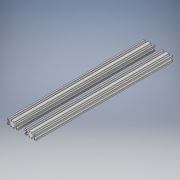
# Autodesk Inventor part: Rail
Saved by Autodesk Inventor 2019 (Build 230136000, 136)
## iProperties
Created: 2021-06-17
Part Number: Rail
Material: Generic
Document SubType Name: Modeling
Designer: 91742
Density: 1 g/cm^3
Appearance: Default
Author: 91742
Autodesk Inventor part; units mm, degrees
ref_plane "YZ Plane" through (0, 0, 0) normal (1, 0, 0) x (0, 1, 0)
ref_plane "XZ Plane" through (0, 0, 0) normal (0, 1, 0) x (-1, 0, 0)
ref_plane "XY Plane" through (0, 0, 0) normal (0, 0, 1) x (1, 0, 0)
sketch "Sketch1" plane through (0, 0, 0) normal (0, 0, 1) x (1, 0, 0)
  circle A0 centre (10, 0) radius 2.1
  line L0 (14.5874, 9.8723) -> (19.0874, 9.8723)
  line L1 (19.0874, 9.8723) -> (14.5874, 9.8723)
  line L2 (14.5874, 9.8723) -> (13.5268, 8.8116)
  line L3 (14.5874, 9.8723) -> (16.0874, 9.8723) construction
  line L4 (13.5268, 8.8116) -> (15.9268, 8.8116)
  line L5 (6.9, 0) -> (6.9, 1.8336)
  line L6 (15.9268, 6.8867) -> (13.1, 4.0599)
  line L7 (15.9268, 8.8116) -> (15.9268, 6.8867)
  line L8 (20.1068, 8.8259) -> (20.1068, 4.3259)
  line L9 (20.1068, 4.3259) -> (19.0461, 3.2652)
  line L10 (19.0461, 3.2652) -> (19.0461, 5.6652)
  line L11 (13.1, 1.8336) -> (16.9316, 5.6652)
  line L12 (19.0461, 5.6652) -> (16.9316, 5.6652)
  line L13 (13.1, 4.0599) -> (6.9, 4.0599)
  line L14 (5.4128, 9.8723) -> (0.9128, 9.8723)
  line L15 (0.9128, 9.8723) -> (5.4128, 9.8723)
  line L16 (5.4128, 9.8723) -> (6.4735, 8.8116)
  line L17 (5.4128, 9.8723) -> (3.9128, 9.8723) construction
  line L18 (4.0732, 6.8867) -> (6.9, 4.0599)
  line L19 (4.0732, 8.8116) -> (4.0732, 6.8867)
  line L20 (6.9, 1.8336) -> (3.0684, 5.6652)
  line L21 (13.1, 0) -> (13.1, 1.8336)
  line L22 (3.0684, 5.6652) -> (3.0684, 8.8116)
  line L23 (3.0684, 8.8116) -> (0.9126, 8.8116)
  circle A1 centre (10, 0) radius 2.1
  line L24 (14.5874, -9.8723) -> (19.0874, -9.8723)
  line L25 (19.0874, -9.8723) -> (14.5874, -9.8723)
  line L26 (14.5874, -9.8723) -> (13.5268, -8.8116)
  line L27 (14.5874, -9.8723) -> (16.0874, -9.8723) construction
  line L28 (13.5268, -8.8116) -> (15.9268, -8.8116)
  line L29 (6.9, 0) -> (6.9, -1.8336)
  line L30 (15.9268, -6.8867) -> (13.1, -4.0599)
  line L31 (15.9268, -8.8116) -> (15.9268, -6.8867)
  line L32 (20.1068, -8.8259) -> (20.1068, -4.3259)
  line L33 (20.1068, -4.3259) -> (19.0461, -3.2652)
  line L34 (19.0461, -3.2652) -> (19.0461, -5.6652)
  line L35 (13.1, -1.8336) -> (16.9316, -5.6652)
  line L36 (19.0461, -5.6652) -> (16.9316, -5.6652)
  line L37 (13.1, -4.0599) -> (6.9, -4.0599)
  line L38 (5.4126, -9.8723) -> (0.9126, -9.8723)
  line L39 (0.9126, -9.8723) -> (5.4126, -9.8723)
  line L40 (5.4126, -9.8723) -> (3.9126, -9.8723) construction
  line L41 (4.0732, -8.8116) -> (4.0732, -6.8867)
  line L42 (6.4732, -8.8116) -> (4.0732, -8.8116)
  line L43 (5.4126, -9.8723) -> (6.4732, -8.8116)
  line L44 (4.0732, -6.8867) -> (6.9, -4.0599)
  line L45 (6.9, -1.8336) -> (3.0684, -5.6652)
  line L46 (13.1, 0) -> (13.1, -1.8336)
  line L47 (3.0684, -5.6652) -> (3.0684, -8.8116)
  line L48 (3.0684, -8.8116) -> (0.9126, -8.8116)
  line L49 (0.9126, 8.8116) -> (-0.2361, 8.8116)
  line L50 (0.9126, -8.8116) -> (-0.2361, -8.8116)
  circle A2 centre (-10, 0) radius 2.1
  line L51 (-14.5874, 9.8723) -> (-19.0874, 9.8723)
  line L52 (-19.0874, 9.8723) -> (-14.5874, 9.8723)
  line L53 (-14.5874, 9.8723) -> (-13.5268, 8.8116)
  line L54 (-14.5874, 9.8723) -> (-16.0874, 9.8723) construction
  line L55 (-13.5268, 8.8116) -> (-15.9277, 8.8116)
  line L56 (-6.9, 0) -> (-6.9, 1.8336)
  line L57 (-15.9072, 6.6932) -> (-13.0532, 3.8939)
  line L58 (-15.9277, 8.8116) -> (-15.9072, 6.6932)
  line L59 (-20.1068, 8.8259) -> (-20.1068, 4.3259)
  line L60 (-20.1068, 4.3259) -> (-19.0461, 3.2652)
  line L61 (-19.0461, 3.2652) -> (-19.0461, 5.6652)
  line L62 (-13.1, 1.8336) -> (-16.9316, 5.6652)
  line L63 (-19.0461, 5.6652) -> (-16.9316, 5.6652)
  line L64 (-13.0532, 3.8939) -> (-6.8535, 3.9539)
  line L65 (-5.4124, 9.8723) -> (-0.9124, 9.8723)
  line L66 (-0.9124, 9.8723) -> (-5.4124, 9.8723)
  line L67 (-5.4124, 9.8723) -> (-3.9124, 9.8723) construction
  line L68 (-4.0736, 8.8116) -> (-4.0542, 6.8079)
  line L69 (-6.473, 8.8116) -> (-4.0736, 8.8116)
  line L70 (-5.4124, 9.8723) -> (-6.473, 8.8116)
  line L71 (-4.0542, 6.8079) -> (-6.8535, 3.9539)
  line L72 (-6.9, 1.8336) -> (-3.0684, 5.6652)
  line L73 (-13.1, 0) -> (-13.1, 1.8336)
  line L74 (-3.0684, 5.6652) -> (-3.0684, 8.8116)
  line L75 (-3.0684, 8.8116) -> (-0.9126, 8.8116)
  line L76 (-4.0732, -6.8867) -> (-6.9, -4.0599)
  line L77 (-6.9, -1.8336) -> (-3.0684, -5.6652)
  line L78 (-6.9, 0) -> (-6.9, -1.8336)
  line L79 (-13.1, -4.0599) -> (-6.9, -4.0599)
  circle A3 centre (-10, 0) radius 2.1
  line L80 (-20.1068, -8.8259) -> (-20.1068, -4.3259)
  line L81 (-20.1068, -4.3259) -> (-19.0461, -3.2652)
  line L82 (-15.9268, -8.8116) -> (-15.9268, -6.8867)
  line L83 (-14.5874, -9.8723) -> (-19.0874, -9.8723)
  line L84 (-19.0874, -9.8723) -> (-14.5874, -9.8723)
  line L85 (-14.5874, -9.8723) -> (-16.0874, -9.8723) construction
  line L86 (-13.5268, -8.8116) -> (-15.9268, -8.8116)
  line L87 (-14.5874, -9.8723) -> (-13.5268, -8.8116)
  line L88 (-3.0684, -5.6652) -> (-3.0684, -8.8116)
  line L89 (-4.0732, -8.8116) -> (-4.0732, -6.8867)
  line L90 (-6.4732, -8.8116) -> (-4.0732, -8.8116)
  line L91 (-3.0684, -8.8116) -> (-0.9126, -8.8116)
  line L92 (-5.4126, -9.8723) -> (-6.4732, -8.8116)
  line L93 (-5.4126, -9.8723) -> (-3.9126, -9.8723) construction
  line L94 (-0.9126, -9.8723) -> (-5.4126, -9.8723)
  line L95 (-5.4126, -9.8723) -> (-0.9126, -9.8723)
  line L96 (-19.0461, -5.6652) -> (-16.9316, -5.6652)
  line L97 (-15.9268, -6.8867) -> (-13.1, -4.0599)
  line L98 (-13.1, -1.8336) -> (-16.9316, -5.6652)
  line L99 (-13.1, 0) -> (-13.1, -1.8336)
  line L100 (-19.0461, -3.2652) -> (-19.0461, -5.6652)
  line L101 (-0.9124, 9.8723) -> (0.2363, 9.8723)
  line L102 (-0.9126, 8.8116) -> (0.2361, 8.8116)
  line L103 (-0.9126, -8.8116) -> (0.2361, -8.8116)
  line L104 (-20.1068, 8.8259) -> (-20.1068, 8.8723)
  line L105 (-19.1068, 9.8723) -> (-19.0874, 9.8723)
  arc A4 (-19.1068, 9.8723) -> (-20.1068, 8.8723) centre (-19.1068, 8.8723) ccw
  line L106 (19.0874, 9.8723) -> (19.1068, 9.8723)
  line L107 (20.1068, 8.8723) -> (20.1068, 8.8259)
  arc A5 (20.1068, 8.8723) -> (19.1068, 9.8723) centre (19.1068, 8.8723) ccw
  line L108 (19.0874, -9.8723) -> (19.1068, -9.8723)
  line L109 (20.1068, -8.8723) -> (20.1068, -8.8116)
  arc A6 (19.1068, -9.8723) -> (20.1068, -8.8723) centre (19.1068, -8.8723) ccw
  line L110 (-20.1068, -8.8259) -> (-20.1068, -8.8723)
  line L111 (-19.1068, -9.8723) -> (-19.0874, -9.8723)
  arc A7 (-20.1068, -8.8723) -> (-19.1068, -9.8723) centre (-19.1068, -8.8723) ccw
  line L112 (-15.9268, -8.8116) -> (-13.5268, -8.8116)
  line L113 (-14.5874, -9.8723) -> (-19.1068, -9.8723)
  line L114 (-20.1068, -8.8723) -> (-20.1068, -4.3259)
  line L115 (-19.0461, -3.2652) -> (-19.0461, -5.6652)
  line L116 (-16.9316, -5.6652) -> (-13.1, -1.8336)
  line L117 (-13.1, 1.8336) -> (-16.9316, 5.6652)
  line L118 (-19.0461, 5.6652) -> (-19.0461, 3.2652)
  line L119 (-20.1068, 4.3259) -> (-20.1068, 8.8404)
  line L120 (-19.1068, 9.8723) -> (-14.5874, 9.8723)
  line L121 (-13.5268, 8.8116) -> (-15.9277, 8.8116)
  line L122 (-15.9072, 6.6932) -> (-13.0532, 3.8939)
  line L123 (-6.8535, 3.9539) -> (-4.0542, 6.8079)
  line L124 (-4.0736, 8.8116) -> (-6.473, 8.8116)
  line L125 (-5.4124, 9.8723) -> (5.4128, 9.8723)
  line L126 (4.0732, 6.8867) -> (6.9, 4.0599)
  line L127 (13.1, 4.0599) -> (15.9268, 6.8867)
  line L128 (15.9268, 8.8116) -> (13.5268, 8.8116)
  line L129 (14.5874, 9.8723) -> (19.1068, 9.8723)
  line L130 (-0.9126, -9.8723) -> (0.9126, -9.8723)
  line L131 (4.0732, 8.8116) -> (6.4735, 8.8116)
  circle A8 centre (75.6379, 0) radius 2.1
  line L132 (80.2253, 9.8723) -> (84.7253, 9.8723)
  line L133 (84.7253, 9.8723) -> (80.2253, 9.8723)
  line L134 (80.2253, 9.8723) -> (79.1646, 8.8116)
  line L135 (80.2253, 9.8723) -> (81.7253, 9.8723) construction
  line L136 (79.1646, 8.8116) -> (81.5646, 8.8116)
  line L137 (72.5379, 0) -> (72.5379, 1.8336)
  line L138 (81.5646, 6.8867) -> (78.7379, 4.0599)
  line L139 (81.5646, 8.8116) -> (81.5646, 6.8867)
  line L140 (85.7446, 8.8259) -> (85.7446, 4.3259)
  line L141 (85.7446, 4.3259) -> (84.684, 3.2652)
  line L142 (84.684, 3.2652) -> (84.684, 5.6652)
  line L143 (78.7379, 1.8336) -> (82.5694, 5.6652)
  line L144 (84.684, 5.6652) -> (82.5694, 5.6652)
  line L145 (78.7379, 4.0599) -> (72.5379, 4.0599)
  line L146 (71.0507, 9.8723) -> (66.5507, 9.8723)
  line L147 (66.5507, 9.8723) -> (71.0507, 9.8723)
  line L148 (71.0507, 9.8723) -> (69.5507, 9.8723) construction
  line L149 (69.7111, 8.8116) -> (69.7111, 6.8867)
  line L150 (71.0507, 9.8723) -> (72.1113, 8.8116)
  line L151 (69.7111, 6.8867) -> (72.5379, 4.0599)
  line L152 (72.5379, 1.8336) -> (68.7063, 5.6652)
  line L153 (78.7379, 0) -> (78.7379, 1.8336)
  line L154 (68.7063, 5.6652) -> (68.7063, 8.8116)
  line L155 (68.7063, 8.8116) -> (66.5504, 8.8116)
  line L156 (69.7111, -6.8867) -> (72.5379, -4.0599)
  line L157 (72.5379, -1.8336) -> (68.7063, -5.6652)
  line L158 (72.5379, 0) -> (72.5379, -1.8336)
  line L159 (78.7379, -4.0599) -> (72.5379, -4.0599)
  circle A9 centre (75.6379, 0) radius 2.1
  line L160 (85.7446, -8.8259) -> (85.7446, -4.3259)
  line L161 (85.7446, -4.3259) -> (84.684, -3.2652)
  line L162 (81.5646, -8.8116) -> (81.5646, -6.8867)
  line L163 (80.2253, -9.8723) -> (84.7253, -9.8723)
  line L164 (84.7253, -9.8723) -> (80.2253, -9.8723)
  line L165 (80.2253, -9.8723) -> (81.7253, -9.8723) construction
  line L166 (79.1646, -8.8116) -> (81.5646, -8.8116)
  line L167 (80.2253, -9.8723) -> (79.1646, -8.8116)
  line L168 (68.7063, -5.6652) -> (68.7063, -8.8116)
  line L169 (69.7111, -8.8116) -> (69.7111, -6.8867)
  line L170 (72.1111, -8.8116) -> (69.7111, -8.8116)
  line L171 (68.7063, -8.8116) -> (66.5504, -8.8116)
  line L172 (71.0504, -9.8723) -> (72.1111, -8.8116)
  line L173 (71.0504, -9.8723) -> (69.5504, -9.8723) construction
  line L174 (66.5504, -9.8723) -> (71.0504, -9.8723)
  line L175 (71.0504, -9.8723) -> (66.5504, -9.8723)
  line L176 (84.684, -5.6652) -> (82.5694, -5.6652)
  line L177 (81.5646, -6.8867) -> (78.7379, -4.0599)
  line L178 (78.7379, -1.8336) -> (82.5694, -5.6652)
  line L179 (78.7379, 0) -> (78.7379, -1.8336)
  line L180 (84.684, -3.2652) -> (84.684, -5.6652)
  line L181 (66.5504, 8.8116) -> (65.4018, 8.8116)
  line L182 (66.5504, -8.8116) -> (65.4018, -8.8116)
  line L183 (45.5311, 8.8259) -> (45.5311, 4.3259)
  line L184 (46.5917, 5.6652) -> (48.7063, 5.6652)
  line L185 (45.5311, 4.3259) -> (46.5917, 3.2652)
  line L186 (46.5917, 3.2652) -> (46.5917, 5.6652)
  line L187 (49.7102, 8.8116) -> (49.7307, 6.6932)
  line L188 (52.1111, 8.8116) -> (49.7102, 8.8116)
  line L189 (51.0504, 9.8723) -> (46.5504, 9.8723)
  line L190 (46.5504, 9.8723) -> (51.0504, 9.8723)
  line L191 (51.0504, 9.8723) -> (49.5504, 9.8723) construction
  line L192 (51.0504, 9.8723) -> (52.1111, 8.8116)
  line L193 (46.5917, -5.6652) -> (48.7063, -5.6652)
  line L194 (45.5311, -8.8259) -> (45.5311, -4.3259)
  line L195 (45.5311, -4.3259) -> (46.5917, -3.2652)
  line L196 (51.0504, -9.8723) -> (46.5504, -9.8723)
  line L197 (46.5504, -9.8723) -> (51.0504, -9.8723)
  line L198 (46.5917, -3.2652) -> (46.5917, -5.6652)
  line L199 (49.7111, -8.8116) -> (49.7111, -6.8867)
  line L200 (52.1111, -8.8116) -> (49.7111, -8.8116)
  line L201 (51.0504, -9.8723) -> (52.1111, -8.8116)
  line L202 (49.7111, -6.8867) -> (52.5379, -4.0599)
  line L203 (52.5379, -1.8336) -> (48.7063, -5.6652)
  line L204 (52.5379, 0) -> (52.5379, -1.8336)
  line L205 (51.0504, -9.8723) -> (49.5504, -9.8723) construction
  line L206 (58.7379, -1.8336) -> (62.5694, -5.6652)
  line L207 (61.5646, -6.8867) -> (58.7379, -4.0599)
  line L208 (59.1646, -8.8116) -> (61.5646, -8.8116)
  line L209 (60.2253, -9.8723) -> (59.1646, -8.8116)
  line L210 (61.5646, -8.8116) -> (61.5646, -6.8867)
  line L211 (62.5694, -5.6652) -> (62.5694, -8.8116)
  line L212 (60.2253, -9.8723) -> (61.7253, -9.8723) construction
  line L213 (64.7253, -9.8723) -> (60.2253, -9.8723)
  line L214 (60.2253, -9.8723) -> (64.7253, -9.8723)
  line L215 (64.7253, -8.8116) -> (65.8739, -8.8116)
  line L216 (62.5694, -8.8116) -> (64.7253, -8.8116)
  line L217 (58.7379, 0) -> (58.7379, 1.8336)
  line L218 (60.2255, 9.8723) -> (64.7255, 9.8723)
  line L219 (64.7255, 9.8723) -> (60.2255, 9.8723)
  line L220 (60.2255, 9.8723) -> (61.7255, 9.8723) construction
  line L221 (61.5642, 8.8116) -> (61.5836, 6.8079)
  line L222 (59.1648, 8.8116) -> (61.5642, 8.8116)
  line L223 (60.2255, 9.8723) -> (59.1648, 8.8116)
  line L224 (61.5836, 6.8079) -> (58.7844, 3.9539)
  line L225 (58.7379, 1.8336) -> (62.5694, 5.6652)
  line L226 (62.5694, 5.6652) -> (62.5694, 8.8116)
  line L227 (62.5694, 8.8116) -> (64.7253, 8.8116)
  line L228 (64.7253, 8.8116) -> (65.8739, 8.8116)
  line L229 (64.7255, 9.8723) -> (65.8741, 9.8723)
  circle A10 centre (55.6379, 0) radius 2.1
  line L230 (49.7307, 6.6932) -> (52.5847, 3.8939)
  line L231 (52.5379, 1.8336) -> (48.7063, 5.6652)
  line L232 (52.5379, 0) -> (52.5379, 1.8336)
  circle A11 centre (55.6379, 0) radius 2.1
  line L233 (52.5379, -4.0599) -> (58.7379, -4.0599)
  line L234 (58.7379, 0) -> (58.7379, -1.8336)
  line L235 (52.5847, 3.8939) -> (58.7844, 3.9539)
  line L236 (45.5311, 8.8259) -> (45.5311, 8.8723)
  line L237 (46.5311, 9.8723) -> (46.5504, 9.8723)
  arc A12 (46.5311, 9.8723) -> (45.5311, 8.8723) centre (46.5311, 8.8723) ccw
  line L238 (84.7253, 9.8723) -> (84.7446, 9.8723)
  line L239 (85.7446, 8.8723) -> (85.7446, 8.8259)
  arc A13 (85.7446, 8.8723) -> (84.7446, 9.8723) centre (84.7446, 8.8723) ccw
  line L240 (84.7253, -9.8723) -> (84.7446, -9.8723)
  line L241 (85.7446, -8.8723) -> (85.7446, -8.8116)
  arc A14 (84.7446, -9.8723) -> (85.7446, -8.8723) centre (84.7446, -8.8723) ccw
  line L242 (45.5311, -8.8259) -> (45.5311, -8.8723)
  line L243 (46.5311, -9.8723) -> (46.5504, -9.8723)
  arc A15 (45.5311, -8.8723) -> (46.5311, -9.8723) centre (46.5311, -8.8723) ccw
  line L244 (49.7111, -8.8116) -> (52.1111, -8.8116)
  line L245 (51.0504, -9.8723) -> (46.5311, -9.8723)
  line L246 (45.5311, -8.8723) -> (45.5311, -4.3259)
  line L247 (46.5917, -3.2652) -> (46.5917, -5.6652)
  line L248 (48.7063, -5.6652) -> (52.5379, -1.8336)
  line L249 (52.5379, 1.8336) -> (48.7063, 5.6652)
  line L250 (46.5917, 5.6652) -> (46.5917, 3.2652)
  line L251 (45.5311, 4.3259) -> (45.5311, 8.8404)
  line L252 (46.5311, 9.8723) -> (51.0504, 9.8723)
  line L253 (52.1111, 8.8116) -> (49.7102, 8.8116)
  line L254 (49.7307, 6.6932) -> (52.5847, 3.8939)
  line L255 (58.7844, 3.9539) -> (61.5836, 6.8079)
  line L256 (61.5642, 8.8116) -> (59.1648, 8.8116)
  line L257 (60.2255, 9.8723) -> (71.0507, 9.8723)
  line L258 (69.7111, 6.8867) -> (72.5379, 4.0599)
  line L259 (78.7379, 4.0599) -> (81.5646, 6.8867)
  line L260 (81.5646, 8.8116) -> (79.1646, 8.8116)
  line L261 (80.2253, 9.8723) -> (84.7446, 9.8723)
  line L262 (64.7253, -9.8723) -> (66.5504, -9.8723)
  line L263 (69.7111, 8.8116) -> (72.1113, 8.8116)
  point P0 (-20.1068, 9.8723)
  point P1 (20.1068, 9.8723)
  point P2 (20.1068, -9.8723)
  point P3 (-20.1068, -9.8723)
  point P4 (45.5311, 9.8723)
  point P5 (85.7446, 9.8723)
  point P6 (85.7446, -9.8723)
  point P7 (45.5311, -9.8723)
  dimension "d0" = 4.2
  dimension "d6" = 4.5
  dimension "d7" = 1.5
  dimension "d8" = 135
  dimension "d9" = 2.4
  dimension "d13" = 3.1
  dimension "d22" = 4.5
  dimension "d23" = 1.5
  dimension "d25" = 2.4
  dimension "d27" = 6.2
  dimension "d29" = 1
  dimension "d30" = 1
  dimension "d31" = 1
  dimension "d32" = 1
  dimension "d33" = 4.2
  dimension "d34" = 4.5
  dimension "d35" = 1.5
  dimension "d36" = 135
  dimension "d37" = 2.4
  dimension "d38" = 3.1
  dimension "d39" = 4.5
  dimension "d40" = 1.5
  dimension "d41" = 2.4
  dimension "d42" = 6.2
  dimension "d43" = 1
  dimension "d44" = 1
  dimension "d45" = 1
  dimension "d46" = 1
  constraints: 528 end point, 32 point on line, 28 collinear, 20 point on circle, 16 centre point, 16 tangent, 14 horizontal, 14 perpendicular, 12 vertical, 2 equal length, 2 parallel
  measures "d0" diameter of A0
  measures "d6" distance of L0.start L0.end
  measures "d7" distance of L0.start L2.end
  measures "d8" angle of L2 L3
  measures "d9" distance of L2.end L4.end
  measures "d13" distance of A0.centre L5.start
  measures "d22" distance of L8.start L8.end
  measures "d23" distance of L8.end L9.end
  measures "d25" distance of L9.end L10.end
  measures "d27" distance of L13.end L6.end
  measures "d29" radius of A4
  measures "d30" radius of A5
  measures "d31" radius of A6
  measures "d32" radius of A7
  measures "d33" diameter of A8
  measures "d34" distance of L132.start L132.end
  measures "d35" distance of L132.start L136.start
  measures "d36" angle of L134 L135
  measures "d37" distance of L136.start L139.start
  measures "d38" distance of A8.centre L137.start
  measures "d39" distance of L239.end L140.end
  measures "d40" distance of L140.end L142.start
  measures "d41" distance of L142.start L144.start
  measures "d42" distance of L151.end L138.end
  measures "d43" radius of A12
  measures "d44" radius of A13
  measures "d45" radius of A14
  measures "d46" radius of A15
extrude "Extrusion1" add sketch "Sketch1" along normal blind 500 contours L0 L106 A5 L107 L8 L9 L10 L12 L11 L21 L46 L35 L36 L34 L33 L32 L109 A6 L108 L24 L26 L28 L31 L30 L37 L44 L41 L42 L43 L38 L130 L94 L92 L90 L89 L76 L79 L97 L82 L86 L87 L83 L111 A7 L110 L80 L81 L100 L96 L98 L99 L73 L62 L63 L61 L60 L59 L104 A4 L105 L51 L53 L55 L58 L57 L64 L71 L68 L69 L70 L65 L101 L125 L14 L16 L131 L19 L18 L13 L6 L7 L4 L2 | L29 L45 L47 L48 L50 L103 L91 L88 L77 L78 L56 L72 L74 L75 L102 L49 L23 L22 L20 L5 | L132 L238 A13 L239 L140 L141 L142 L144 L143 L153 L179 L178 L176 L180 L161 L160 L241 A14 L240 L163 L167 L166 L162 L177 L159 L156 L169 L170 L172 L174 L262 L213 L209 L208 L210 L207 L233 L202 L199 L200 L201 L196 L243 A15 L242 L194 L195 L198 L193 L203 L204 L232 L231 L184 L186 L185 L183 L236 A12 L237 L189 L192 L188 L187 L230 L235 L224 L221 L222 L223 L218 L229 L257 L146 L150 L263 L149 L151 L145 L138 L139 L136 L134 | L158 L157 L168 L171 L182 L215 L216 L211 L206 L234 L217 L225 L226 L227 L228 L181 L155 L154 L152 L137
body "Solid1"
